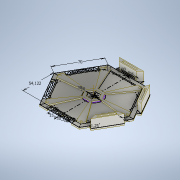
# Autodesk Inventor part: HexagoneBack
Saved by Autodesk Inventor 2020 (Build 240168000, 168)
## iProperties
Created: 2020-04-08
Part Number: HexagoneBack
Material: Silver
Document SubType Name: Modeling
Designer: Samuele
Density: 10.49 g/cm^3
Appearance: Silver
Author: Samuele
Autodesk Inventor part; units mm, degrees
ref_plane "YZ Plane" through (0, 0, 0) normal (1, 0, 0) x (0, 1, 0)
ref_plane "XZ Plane" through (0, 0, 0) normal (0, 1, 0) x (-1, 0, 0)
ref_plane "XY Plane" through (0, 0, 0) normal (0, 0, 1) x (1, 0, 0)
sketch "Sketch6" plane through (0, 0, 0) normal (0, 1, 0) x (-1, 0, 0)
  line L0 (102.5, -48.5) -> (-37.5, -48.5)
  line L1 (32.5, -118.5) -> (32.5, 21.5)
  line L2 (102.5, -48.5) -> (67.5, -109.1218)
  line L3 (67.5, -109.1218) -> (-2.5, -109.1218)
  line L4 (-2.5, -109.1218) -> (-37.5, -48.5)
  line L5 (-37.5, -48.5) -> (-2.5, 12.1218)
  line L6 (-2.5, 12.1218) -> (67.5, 12.1218)
  line L7 (67.5, 12.1218) -> (102.5, -48.5)
  line L8 (32.5, 12.1218) -> (85, -18.1891)
  line L9 (85, -18.1891) -> (85, -78.8109)
  line L10 (85, -78.8109) -> (32.5, -109.1218)
  line L11 (32.5, -109.1218) -> (-20, -78.8109)
  line L12 (-20, -78.8109) -> (-20, -18.1891)
  line L13 (-20, -18.1891) -> (32.5, 12.1218)
  line L14 (32.5, 12.1218) -> (47.5, 12.1218)
  line L15 (47.5, 12.1218) -> (47.5, 5.6218)
  line L16 (47.5, 5.6218) -> (17.5, 5.6218)
  line L17 (17.5, 5.6218) -> (17.5, 12.1218)
  line L18 (47.5, 5.6218) -> (56.6924, 5.6218) construction
  line L19 (17.5, 8.8718) -> (20, 8.8718)
  line L20 (47.5, 8.8718) -> (45, 8.8718)
  line L21 (45, 8.8718) -> (45, 10.1218)
  line L22 (45, 10.1218) -> (20, 10.1218)
  line L23 (20, 10.1218) -> (20, 7.6218)
  line L24 (20, 7.6218) -> (45, 7.6218)
  line L25 (45, 7.6218) -> (45, 10.1218)
  line L26 (67.5, 12.1218) -> (32.5, -48.5)
  line L27 (32.5, -48.5) -> (67.5, -109.1218)
  line L28 (47.5, 5.6218) -> (56.6924, 5.6218)
  line L29 (17.5, 5.6218) -> (11, 5.6218)
  line L30 (17.5, 12.1218) -> (11, 5.6218)
  line L31 (17.5, 12.1218) -> (26.6924, 12.1218) construction
  line L32 (47.5, 12.1218) -> (54, 5.6218)
  line L33 (85, -18.1891) -> (77.5, -5.1987)
  line L34 (77.5, -5.1987) -> (71.8708, -8.4487)
  line L35 (71.8708, -8.4487) -> (86.8708, -34.4295)
  line L36 (86.8708, -34.4295) -> (92.5, -31.1795)
  line L37 (71.8708, -8.4487) -> (67.2746, -0.4879) construction
  line L38 (89.6854, -32.8045) -> (88.4354, -30.6394)
  line L39 (74.6854, -6.8237) -> (75.9354, -8.9888)
  line L40 (75.9354, -8.9888) -> (77.0179, -8.3638)
  line L41 (77.0179, -8.3638) -> (89.5179, -30.0144)
  line L42 (89.5179, -30.0144) -> (87.3529, -31.2644)
  line L43 (87.3529, -31.2644) -> (74.8529, -9.6138)
  line L44 (74.8529, -9.6138) -> (77.0179, -8.3638)
  line L45 (71.8708, -8.4487) -> (67.2746, -0.4879)
  line L46 (86.8708, -34.4295) -> (90.1208, -40.0587)
  line L47 (92.5, -31.1795) -> (90.1208, -40.0587)
  line L48 (92.5, -31.1795) -> (87.9038, -23.2187) construction
  line L49 (77.5, -5.1987) -> (68.6208, -2.8196)
  line L50 (71.8708, -88.5513) -> (67.2746, -96.5121) construction
  line L51 (74.6854, -90.1763) -> (75.9354, -88.0112)
  line L52 (74.8529, -87.3862) -> (77.0179, -88.6362)
  line L53 (77.5, -91.8013) -> (71.8708, -88.5513)
  line L54 (77.5, -91.8013) -> (68.6208, -94.1804)
  line L55 (71.8708, -88.5513) -> (67.2746, -96.5121)
  line L56 (77.0179, -88.6362) -> (89.5179, -66.9856)
  line L57 (87.3529, -65.7356) -> (74.8529, -87.3862)
  line L58 (71.8708, -88.5513) -> (86.8708, -62.5705)
  line L59 (89.5179, -66.9856) -> (87.3529, -65.7356)
  line L60 (89.6854, -64.1955) -> (88.4354, -66.3606)
  line L61 (86.8708, -62.5705) -> (92.5, -65.8205)
  line L62 (86.8708, -62.5705) -> (90.1208, -56.9413)
  line L63 (92.5, -65.8205) -> (90.1208, -56.9413)
  line L64 (94.9944, -48.5) -> (63.7472, -102.6218)
  line L65 (-29.9944, -48.5) -> (1.2528, 5.6218)
  line L66 (1.2528, 5.6218) -> (63.7472, 5.6218)
  line L67 (63.7472, 5.6218) -> (94.9944, -48.5)
  line L68 (32.5, -109.1218) -> (32.5, -115.6218)
  line L69 (32.5, -115.6218) -> (54, -115.6218)
  line L70 (47.5, -115.6218) -> (47.5, -109.1218)
  line L71 (47.5, -109.1218) -> (54, -115.6218)
  line L72 (32.5, -115.6218) -> (11, -115.6218)
  line L73 (17.5, -115.6218) -> (17.5, -109.1218)
  line L74 (17.5, -109.1218) -> (11, -115.6218)
  line L75 (54, -115.6218) -> (54, -109.1218)
  line L76 (11, -115.6218) -> (11, -109.1218)
  line L77 (90.1208, -40.0587) -> (95.75, -36.8087)
  line L78 (68.6208, -2.8196) -> (74.25, 0.4304)
  line L79 (90.1208, -56.9413) -> (95.75, -60.1913)
  line L80 (68.6208, -94.1804) -> (74.25, -97.4304)
  line L81 (11, 5.6218) -> (11, 12.1218)
  line L82 (54, 5.6218) -> (54, 12.1218)
  line L83 (32.5, -109.1218) -> (32.5, -111.1218)
  line L84 (32.5, -111.1218) -> (45, -111.1218)
  line L85 (45, -111.1218) -> (45, -113.6218)
  line L86 (45, -113.6218) -> (20, -113.6218)
  line L87 (20, -113.6218) -> (20, -111.1218)
  line L88 (20, -111.1218) -> (32.5, -111.1218)
  line L89 (32.5, -48.5) -> (-2.5, -109.1218)
  line L90 (32.5, -48.5) -> (-2.5, 12.1218)
  line L91 (-20, -78.8109) -> (-25.6292, -82.0609)
  line L92 (-25.6292, -82.0609) -> (-36.3792, -63.4413)
  line L93 (-33.1292, -69.0705) -> (-27.5, -65.8205)
  line L94 (-27.5, -65.8205) -> (-36.3792, -63.4413)
  line L95 (-25.6292, -82.0609) -> (-14.8792, -100.6804)
  line L96 (-18.1292, -95.0513) -> (-12.5, -91.8013)
  line L97 (-12.5, -91.8013) -> (-14.8792, -100.6804)
  line L98 (-36.3792, -63.4413) -> (-30.75, -60.1913)
  line L99 (-14.8792, -100.6804) -> (-9.25, -97.4304)
  line L100 (-20, -78.8109) -> (-21.7321, -79.8109)
  line L101 (-21.7321, -79.8109) -> (-27.9821, -68.9856)
  line L102 (-27.9821, -68.9856) -> (-30.1471, -70.2356)
  line L103 (-30.1471, -70.2356) -> (-17.6471, -91.8862)
  line L104 (-17.6471, -91.8862) -> (-15.4821, -90.6362)
  line L105 (-15.4821, -90.6362) -> (-21.7321, -79.8109)
  line L106 (-20, -18.1891) -> (-25.6292, -14.9391)
  line L107 (-25.6292, -14.9391) -> (-36.3792, -33.5587)
  line L108 (-33.1292, -27.9295) -> (-27.5, -31.1795)
  line L109 (-27.5, -31.1795) -> (-36.3792, -33.5587)
  line L110 (-25.6292, -14.9391) -> (-14.8792, 3.6804)
  line L111 (-18.1292, -1.9487) -> (-12.5, -5.1987)
  line L112 (-15.4821, -6.3638) -> (-21.7321, -17.1891)
  line L113 (-20, -18.1891) -> (-21.7321, -17.1891)
  line L114 (-21.7321, -17.1891) -> (-27.9821, -28.0144)
  line L115 (-14.8792, 3.6804) -> (-9.25, 0.4304)
  line L116 (-12.5, -5.1987) -> (-14.8792, 3.6804)
  line L117 (-36.3792, -33.5587) -> (-30.75, -36.8087)
  line L118 (-17.6471, -5.1138) -> (-15.4821, -6.3638)
  line L119 (-27.9821, -28.0144) -> (-30.1471, -26.7644)
  line L120 (-30.1471, -26.7644) -> (-17.6471, -5.1138)
  line L121 (-29.0646, -27.3894) -> (-30.3146, -29.5545)
  line L122 (-29.0646, -69.6106) -> (-30.3146, -67.4455)
  line L123 (-16.5646, -91.2612) -> (-15.3146, -93.4263)
  line L124 (20, -112.3718) -> (17.5, -112.3718)
  line L125 (45, -112.3718) -> (47.5, -112.3718)
  line L126 (-15.3146, -3.5737) -> (-16.5646, -5.7388)
  line L127 (20, -111.1218) -> (20, -109.1218)
  line L128 (45, -111.1218) -> (45, -109.1218)
  line L129 (-15.4821, -90.6362) -> (-13.75, -89.6362)
  line L130 (-27.9821, -68.9856) -> (-26.25, -67.9856)
  line L131 (-15.4821, -6.3638) -> (-13.75, -7.3638)
  line L132 (-27.9821, -28.0144) -> (-26.25, -29.0144)
  line L133 (63.7472, -102.6218) -> (1.2528, -102.6218)
  line L134 (1.2528, -102.6218) -> (-29.9944, -48.5)
  line L135 (-29.9944, -48.5) -> (1.2528, 5.6218)
  line L136 (1.2528, 5.6218) -> (63.7472, 5.6218)
  line L137 (63.7472, 5.6218) -> (94.9944, -48.5)
  line L138 (94.9944, -48.5) -> (63.7472, -102.6218)
  line L139 (-29.9944, -48.5) -> (-27.9944, -48.5)
  line L140 (-27.9944, -48.5) -> (2.2528, 3.8897)
  line L141 (2.2528, 3.8897) -> (62.7472, 3.8897)
  line L142 (62.7472, 3.8897) -> (92.9944, -48.5)
  line L143 (92.9944, -48.5) -> (62.7472, -100.8897)
  line L144 (62.7472, -100.8897) -> (2.2528, -100.8897)
  line L145 (2.2528, -100.8897) -> (-27.9944, -48.5)
  line L146 (32.5, -48.5) -> (56.7472, -102.6218)
  line L147 (32.5, -48.5) -> (67.2472, -96.5596)
  line L148 (62.7472, -100.8897) -> (60.7472, -97.4256)
  line L149 (60.7472, -97.4256) -> (66.1352, -95.0216)
  line L150 (60.7472, -97.4256) -> (55.9712, -100.8897)
  line L151 (63.7472, -102.6218) -> (62.2472, -100.0237)
  circle A0 centre (62.2472, -100.0237) radius 1.5
  circle A1 centre (32.5, -48.5) radius 10
  circle A2 centre (32.5, -48.5) radius 15
  line L152 (22.5, -48.5) -> (27.5, -39.8397)
  line L153 (27.5, -39.8397) -> (37.5, -39.8397)
  line L154 (37.5, -39.8397) -> (42.5, -48.5)
  line L155 (42.5, -48.5) -> (37.5, -57.1603)
  line L156 (37.5, -57.1603) -> (27.5, -57.1603)
  line L157 (27.5, -57.1603) -> (22.5, -48.5)
  line L158 (17.5, -48.5) -> (25, -35.5096)
  line L159 (25, -35.5096) -> (40, -35.5096)
  line L160 (40, -35.5096) -> (47.5, -48.5)
  line L161 (47.5, -48.5) -> (40, -61.4904)
  line L162 (40, -61.4904) -> (25, -61.4904)
  line L163 (25, -61.4904) -> (17.5, -48.5)
  circle A3 centre (32.5, -48.5) radius 3.5
  line L164 (32.5, -48.5) -> (26.5, -48.5)
  circle A4 centre (26.5, -48.5) radius 2
  line L165 (26.5, -46.5) -> (29.6277, -46.5)
  line L166 (26.5, -50.5) -> (29.6277, -50.5)
  point P0 (32.5, -48.5)
  point P1 (63.6096, -99.3961)
  point P2 (61.0225, -100.8897)
  point P3 (40.8401, -60.0353)
  point P4 (38.3591, -56.6038)
  point P5 (38.06, -56.1902)
  point P6 (36.3799, -57.1603)
  dimension "d142" = 20
  dimension "d143" = 30
  dimension "d87" = 15
  dimension "d88" = 6.5
  dimension "d91" = 2.5
  dimension "d92" = 2.5
  dimension "d95" = 1.25
  dimension "d96" = 25
  dimension "d97" = 2.5
  dimension "d98" = 25
  dimension "d99" = 135
  dimension "d100" = 0
  dimension "d105" = 30
  dimension "d108" = 6.5
  dimension "d111" = 45
  dimension "d112" = 15
  dimension "d113" = 2
  dimension "d114" = 12.5
  dimension "d115" = 2.5
  dimension "d116" = 25
  dimension "d118" = 70
  dimension "d119" = 54.1218
  dimension "d120" = 1.25
  dimension "d127" = 2
  dimension "d130" = 7
  dimension "d136" = 4
  dimension "d138" = 3
  dimension "d139" = 3
  dimension "d144" = 7
  dimension "d145" = 6
  dimension "d146" = 4
  constraints: 334 end point, 77 symmetric about line, 36 point on line, 17 midpoint, 13 perpendicular, 12 coincident, 9 horizontal, 4 point on circle, 3 centre point, 2 collinear, 2 horizontal alignment, 2 tangent, 2 vertical, 1 equal length, 1 parallel, 95 other
  measures "d87" distance of L8.start L14.end
  measures "d88" distance of L14.end L15.end
  measures "d91" distance of L19.start L19.end
  measures "d92" distance of L20.start L20.end
  measures "d95" distance of L20.end L21.end
  measures "d96" distance of L21.end L22.end
  measures "d97" distance of L22.end L23.end
  measures "d98" distance of L23.end L24.end
  measures "d99" angle of L30 L31
  measures "d100" distance of L17.end L30.start
  measures "d105" distance of L17.end L14.end
  measures "d108" distance of L10.end L68.end
  measures "d111" angle of L70 L71
  measures "d112" distance between parallel lines of L68 L70
  measures "d113" distance of L10.end L83.end
  measures "d114" distance of L83.end L84.end
  measures "d115" distance of L84.end L85.end
  measures "d116" distance of L85.end L86.end
  measures "d118" distance of L0.start L2.end
  measures "d119" vertical distance of L66.end L64.start
  measures "d120" vertical distance of L118.start L118.end
  measures "d127" distance of L134.end L139.end
  measures "d130" distance of L146.end L64.end
  measures "d136" distance of L143.end L148.end
  measures "d138" distance of L64.end L151.end
  measures "d139" diameter of A0
  measures "d144" diameter of A3
  measures "d145" distance of L164.start L164.end
  measures "d146" diameter of A4
extrude "Plate" add sketch "Sketch6" against normal blind 3 contours L2 L79 L64 L0 | L0 L67 L77 L7 | L64 L62 L58 L9 L143 L0 | L0 L142 L9 L35 L46 L67 | L143 L9 L0 | L0 L9 L142 | L9 L143 L10 L147 A2 L0 | L0 A2 L26 L8 L142 L9 | L142 L8 L35 L9 | L9 L58 L10 L143 | L161 L147 A1 L0 | L160 A2 | L0 A1 L26 L160 | A2 L147 L161 | L142 L26 L67 L45 L35 L8 | L8 L26 L142 | L143 L147 L10 | L10 L58 L55 L64 L147 L143 | L155 L147 A3 L0 | L154 A1 | L0 A3 L26 L154 | A1 L147 L155 | A2 L1 L141 L8 L26 | L159 L1 A2 | L26 A1 L1 L159 | A2 L161 L147 | L147 L10 L27 A2 | L161 L27 A1 L147 | L8 L141 L26 | L141 L8 L16 L28 L66 L26 | L147 L149 L27 L10 | L147 L64 L27 A0 L143 | L143 A0 L27 L149 | L2 L27 L64 L55 L80 | L78 L45 L67 L26 L7 | A3 L147 L0 | L0 L26 A3 | L153 L1 A1 | L26 A3 L1 L153 | A1 L155 L147 | L155 L27 A3 L147 | A2 L90 L13 L141 L1 | L1 L159 A2 | L1 A1 L90 L159 | L162 L146 A1 L27 | L27 L10 L146 A2 | A2 L146 L162 | L141 L1 L16 L8 | L66 L28 L82 L6 L26 | L27 L150 L146 L10 | A0 L27 L143 | L143 L27 A0 | L27 A0 L144 L150 | L3 L10 L133 L27 | L89 A3 L0 | L146 A3 L1 | L90 A3 L1 | L1 A3 L26 | L147 A3 L27 | L1 A3 L89 | L0 A3 L90 | L27 A3 L146 | L1 L153 A1 | L1 A3 L90 L153 | L156 L146 A3 L27 | A1 L146 L156 | L141 L13 L16 L1 | A2 L0 L12 L140 L13 L90 | L158 A2 | L90 A1 L0 L158 | A2 L1 L162 L146 | L146 L10 L144 L1 A2 | L162 L1 A1 L146 | L146 L144 L10 | L144 A0 L27 | L27 A0 L144 | L133 L146 L144 A0 L27 | L146 L133 L10 L144 | L75 L71 L3 | A3 L166 A4 L0 | L0 A4 L165 A3 | A3 L146 L156 L1 | L1 L156 L89 A3 | L89 L157 L0 A4 L166 A3 | A3 L165 A4 L0 L152 L90 | L152 A1 | A1 L1 L156 L146 | L141 L90 L66 L29 L16 L13 | L13 L90 L141 | L13 L140 L90 | A2 L89 L11 L145 L12 L0 | L163 A2 | L0 A1 L89 L163 | A2 L162 L1 | L1 L144 L11 L89 A2 | L162 L89 A1 L1 | L10 L133 L1 L144 | L70 L125 L85 L128 L3 | L71 L69 L70 | A4 L0 | L0 A4 | L1 A1 L156 | A1 L157 | L140 L13 L65 L90 | L140 L12 L65 L13 | L12 L145 L0 | L0 L140 L12 | L1 L133 L11 L144 | L10 L1 L133 | L128 L84 L1 L3 | L70 L69 L1 L86 L85 L125 | L90 L6 L81 L66 | L65 L13 L5 L90 | L65 L12 L13 | L140 L0 L65 L12 | L145 L12 L134 L0 | L145 L11 L134 L12 | L89 L145 L11 | L11 L144 L89 | L1 L11 L133 | L11 L133 L89 L144 | L1 L88 L127 L3 | L3 L89 L133 L11 | L85 L86 L1 L84 | L72 L73 L124 L87 L86 L1 | L12 L65 L0 L5 | L106 L112 L131 L5 | L5 L132 L114 L106 | L134 L12 L4 L0 | L134 L11 L12 | L145 L89 L134 L11 | L1 L86 L87 L88 | L127 L87 L124 L73 L3 | L72 L74 L73 | L5 L116 L115 | L5 L108 L121 L119 L132 | L131 L118 L126 L111 L5 | L114 L119 L120 L106 | L106 L120 L118 L112 | L11 L134 L89 L4 | L91 L101 L130 L4 | L4 L129 L105 L91 | L74 L76 L3 | L111 L110 L116 | L109 L107 L108 | L5 L117 L109 | L120 L119 L121 L108 L107 L106 | L106 L110 L111 L126 L118 L120 | L4 L94 L98 | L4 L96 L123 L104 L129 | L130 L102 L122 L93 L4 | L105 L104 L103 L91 | L91 L103 L102 L101 | L93 L92 L94 | L97 L95 L96 | L4 L99 L97 | L103 L104 L123 L96 L95 L91 | L91 L92 L93 L122 L102 L103
extrude "Cazzetti" add sketch "Sketch6" along normal blind 15 contours L70 L125 L85 L128 L3 | L71 L69 L70 | L128 L84 L1 L3 | L70 L69 L1 L86 L85 L125 | L1 L88 L127 L3 | L72 L73 L124 L87 L86 L1 | L106 L112 L131 L5 | L5 L132 L114 L106 | L127 L87 L124 L73 L3 | L72 L74 L73 | L5 L108 L121 L119 L132 | L131 L118 L126 L111 L5 | L91 L101 L130 L4 | L4 L129 L105 L91 | L111 L110 L116 | L109 L107 L108 | L120 L119 L121 L108 L107 L106 | L106 L110 L111 L126 L118 L120 | L4 L96 L123 L104 L129 | L130 L102 L122 L93 L4 | L93 L92 L94 | L97 L95 L96 | L103 L104 L123 L96 L95 L91 | L91 L92 L93 L122 L102 L103
extrude "ScavoStrip" cut sketch "Sketch6" along normal blind 5 contours L128 L84 L1 L3 | L1 L88 L127 L3 | L106 L112 L131 L5 | L5 L132 L114 L106 | L91 L101 L130 L4 | L4 L129 L105 L91
extrude "ScalinoAllineamento" add sketch "Sketch6" along normal blind 2 contours L161 L147 A1 L0 | A1 L147 L155 | A2 L161 L147 | L147 L10 L27 A2 | L161 L27 A1 L147 | L147 L149 L27 L10 | L147 L64 L27 A0 L143 | L143 A0 L27 L149 | A1 L155 L147 | L162 L146 A1 L27 | L27 L10 L146 A2 | A2 L146 L162 | L27 L150 L146 L10 | L27 A0 L144 L150 | A1 L146 L156 | L133 L146 L144 A0 L27 picked at (40.4263, -60.9175)
extrude "Foro" cut sketch "Sketch6" against normal blind 9.25 contours A0 L27 L143 | L143 L27 A0 | L144 A0 L27 | L27 A0 L144
pattern_circular "ScalinoCircolare" count 6 over 360 about axis through (-32.5, 0, -48.5) along (0, 1, 0) of "ScalinoAllineamento", "Foro"
extrude "Extrusion15" cut sketch "Sketch6" against normal blind 10 contours A3 L147 L0 | L0 L26 A3 | L89 A3 L0 | L146 A3 L1 | L90 A3 L1 | L1 A3 L26 | L147 A3 L27 | L1 A3 L89 | L0 A3 L90 | L27 A3 L146 | A3 L166 A4 L0 | L0 A4 L165 A3 | A4 L0 | L0 A4
body "Solid4"
